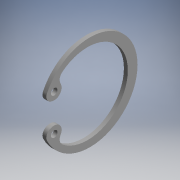
# Autodesk Inventor part: RTWN28
Saved by Autodesk Inventor 2017.3 (Build 213256000, 256)
## iProperties
Part Number: RTWN28
Material: Generic
Catalog Web Link: www.cadenas.de
Description: RTWN, RTWS-Retaining Rings - C - Internal
Vendor: MISUMI
Document SubType Name: Modeling
Designer: partserver
Manufacturer: MISUMI
Mass: 0.23542 g
Surface Area: 5.99729 cm^2
Volume: 0.23542 cm^3
Density: 1 g/cm^3
Appearance: PSOLRGB-192-192-192
Category: PARTsolutions
Company: MISUMI
Title: RTWN28
Author: Cadenas PARTsolutions
Comments: Retaining Rings - C - Internal
PSOL_IDENT_0: {$CADENAS_DATA\23d-libs\misumi\metric\28_keys_magnets\rtwn.prj},160 {VTYP=3D},{NB=RTWN28},{LINA=RTWN
PSOL_IDENT_1: 28},{NN=RTWN, RTWS},{DATE=30.06.2021 13:10:00},{GEOMDATE=31.07.2012 00:00:00},{VERSION=},{LINEID=150
PSOL_IDENT_2: },{WBVAR=MAT},{WBNUMERIC=}  {NB=RTWN28},{LINA=RTWN28},{KT=DUMMY},{PN=RTWN28},{TYPE=RTWN},{MAT=1},{HA
PSOL_IDENT_3: RD=44~53HRC},{NO=28},{DD3=30.1},{DD3TOL=+0.25/-0.25},{TT=1.20},{TTTOL=+0.06/-0.06},{BB=3.0},{AA=4.6}
PSOL_IDENT_4: ,{DD0=2.0},{DD4=18},{DD1=28},{DD2=29.4},{DD2TOL=+0.21/0},{MM=1.35},{MMTOL=+0.14/0},{NN=1.5},{A2=11.3
PSOL_IDENT_5: 0}
NB: RTWN28
NN: 1.5
NT: Retaining Rings - C - Internal
NBSYN: $PN.
LINA: RTWN28
CATALOG: Misumi
PN: RTWN28
MAT: Spring Steel
HARD: 44~53HRC
NO: 28
DD3: 30.1
DD3TOL: +0.25/-0.25
TT: 1.2
TTTOL: +0.06/-0.06
BB: 3
AA: 4.6
DD0: 2
DD4: 18
DD1: 28
DD2: 29.4
DD2TOL: +0.21/0
MM: 1.35
MMTOL: +0.14/0
SUPPLIER: MISUMI
ARTICLENO: RTWN28
BOMINFO: RTWN28
CREATOR: CADENAS GmbH
Autodesk Inventor part; units mm, degrees
sketch "Sketch_3" plane through (0, 0, 0) normal (1, 0, 0) x (0, 1, 0)
  arc A0 (-13.2705, -6.3234) -> (-13.2705, 6.3234) centre (0, 0) ccw
  arc A1 (-13.2705, 6.3234) -> (-12.0302, 3.5446) centre (-11.465, 5.463) ccw
  line L0 (-12.0302, 3.5446) -> (-11.688, 3.4438)
  arc A2 (-11.688, 3.4438) -> (-9.0471, 6.8016) centre (-11.038, 5.65) ccw
  arc A3 (-8.4852, 9.7555) -> (-9.0471, 6.8016) centre (-7.0562, 7.9533) ccw
  arc A4 (-8.4852, -9.7555) -> (-8.4852, 9.7555) centre (-0.75, 0) ccw
  arc A5 (-9.0471, -6.8016) -> (-8.4852, -9.7555) centre (-7.0562, -7.9533) ccw
  arc A6 (-9.0471, -6.8016) -> (-11.688, -3.4438) centre (-11.038, -5.65) ccw
  line L1 (-11.688, -3.4438) -> (-12.0302, -3.5446)
  arc A7 (-12.0302, -3.5446) -> (-13.2705, -6.3234) centre (-11.465, -5.463) ccw
  circle A8 centre (-11.038, -5.65) radius 1
  circle A9 centre (-11.038, 5.65) radius 1
  constraints: 16 point on circle, 10 centre point, 4 end point
extrude "Extrusion1" add sketch "Sketch_3" along normal mid plane 1.2
ref_plane "rr_XY" through (-0.6, 0, 0) normal (1, 0, 0) x (0, 0, -1)
ref_plane "rr_YZ" through (-0.6, 0, 0) normal (0, 0, -1) x (0, 1, 0)
ref_plane "rr_ZX" through (-0.6, 0, 0) normal (0, 1, 0) x (1, 0, 0)
body "Solid1"
